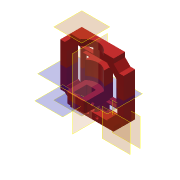
# Autodesk Inventor part: 20_Cube_Inser_Flexuremanipulator_ST_connector_zonly_v3
Saved by Autodesk Inventor 2019.4 (Build 234330000, 330)
## iProperties
Created: 2019-07-01
Part Number: 20_Cube_Inser_Flexuremanipulator_ST_connector_zonly_v3
Material: Generic
Document SubType Name: Modeling
Designer: diederichbenedict
Density: 1 g/cm^3
Appearance: Light Red
Author: diederichbenedict
Autodesk Inventor part; units mm, degrees
ref_plane "YZ Plane" through (0, 0, 0) normal (1, 0, 0) x (0, 1, 0)
ref_plane "XZ Plane" through (0, 0, 0) normal (0, 1, 0) x (-1, 0, 0)
ref_plane "Work Plane1" through (0, 0, 10) normal (0, 0, 1) x (1, 0, 0)
ref_plane "Work Plane4" through (0, 0, 13) normal (0, 0, 1) x (1, 0, 0)
sketch "Sketch5" plane through (0, 0, 13) normal (0, 0, 1) x (1, 0, 0)
  line L0 (-3.9299, 45.8299) -> (-37.9299, 45.8299) projected
  line L1 (-37.9299, 45.8299) -> (-37.9299, 42.2551) projected
  line L2 (-37.9299, 42.2551) -> (-42.2551, 37.9299) projected
  line L3 (-42.2551, 37.9299) -> (-45.8299, 37.9299) projected
  line L4 (-45.8299, 37.9299) -> (-45.8299, 3.9299) projected
  line L5 (-42.2551, 3.9299) -> (-45.8299, 3.9299) projected
  line L6 (-37.9299, -0.3953) -> (-42.2551, 3.9299) projected
  line L7 (-37.9299, -3.9701) -> (-37.9299, -0.3953) projected
  line L8 (-3.9713, -3.9701) -> (-37.9299, -3.9701) projected
  line L9 (-3.9713, -3.9701) -> (-3.9713, -0.4367) projected
  line L10 (-3.9713, -0.4367) -> (0.3953, 3.9299) projected
  line L11 (0.3953, 3.9299) -> (3.9701, 3.9299) projected
  line L12 (3.9701, 3.9299) -> (3.9701, 37.9299) projected
  line L13 (3.9701, 37.9299) -> (0.3953, 37.9299) projected
  line L14 (0.3953, 37.9299) -> (-3.9299, 42.2551) projected
  line L15 (-3.9299, 42.2551) -> (-3.9299, 45.8299) projected
  line L16 (-1.0299, 32.9299) -> (-1.0299, 8.9299)
  line L17 (-1.0299, 8.9299) -> (-1.6758, 8.9299)
  line L18 (-1.6758, 8.9299) -> (-8.9713, 1.6344)
  line L19 (-8.9713, 1.6344) -> (-8.9713, 1.0299)
  line L20 (-8.9713, 1.0299) -> (-32.9299, 1.0299)
  line L21 (-32.9299, 1.0299) -> (-32.9299, 1.6758)
  line L22 (-32.9299, 1.6758) -> (-40.184, 8.9299)
  line L23 (-40.184, 8.9299) -> (-40.8299, 8.9299)
  line L24 (-40.8299, 8.9299) -> (-40.8299, 32.9299)
  line L25 (-40.8299, 32.9299) -> (-40.184, 32.9299)
  line L26 (-40.184, 32.9299) -> (-32.9299, 40.184)
  line L27 (-32.9299, 40.184) -> (-32.9299, 40.8299)
  line L28 (-32.9299, 40.8299) -> (-8.9299, 40.8299)
  line L29 (-8.9299, 40.8299) -> (-8.9299, 40.184)
  line L30 (-8.9299, 40.184) -> (-1.6758, 32.9299)
  line L31 (-1.6758, 32.9299) -> (-1.0299, 32.9299)
  dimension "d46" = 5
  constraints: 32 end point, 15 other
  measures "d46" distance between parallel lines of L12 L16
extrude "Extrusion5" add sketch "Sketch5" along normal blind 6 and the other way blind 3
ref_plane "Work Plane5" through (0, 0, 21) normal (0, 0, 1) x (1, 0, 0)
sketch "Sketch7" plane through (0, 0, 10) normal (0, 0, 1) x (1, 0, 0)
  line L0 (-1.0299, 8.9299) -> (-1.6758, 8.9299) projected
  line L1 (-1.6758, 8.9299) -> (-8.9713, 1.6344) projected
  line L2 (-8.9713, 1.6344) -> (-8.9713, 1.0299) projected
  line L3 (-8.9713, 1.0299) -> (-32.9299, 1.0299) projected
  line L4 (-32.9299, 1.0299) -> (-32.9299, 1.6758) projected
  line L5 (-32.9299, 1.6758) -> (-40.184, 8.9299) projected
  line L6 (-40.184, 8.9299) -> (-40.8299, 8.9299) projected
  line L7 (-40.8299, 8.9299) -> (-40.8299, 32.9299) projected
  line L8 (-40.8299, 32.9299) -> (-40.184, 32.9299) projected
  line L9 (-40.184, 32.9299) -> (-32.9299, 40.184) projected
  line L10 (-32.9299, 40.184) -> (-32.9299, 40.8299) projected
  line L11 (-32.9299, 40.8299) -> (-8.9299, 40.8299) projected
  line L12 (-8.9299, 40.8299) -> (-8.9299, 40.184) projected
  line L13 (-8.9299, 40.184) -> (-1.6758, 32.9299) projected
  line L14 (-1.6758, 32.9299) -> (-1.0299, 32.9299) projected
  line L15 (-1.0299, 32.9299) -> (-1.0299, 8.9299) projected
  line L16 (-3.9299, 45.8299) -> (-37.9299, 45.8299) projected
  line L17 (-37.9299, 45.8299) -> (-37.9299, 42.2551) projected
  line L18 (-37.9299, 42.2551) -> (-42.2551, 37.9299) projected
  line L19 (-42.2551, 37.9299) -> (-45.8299, 37.9299) projected
  line L20 (-45.8299, 37.9299) -> (-45.8299, 3.9299) projected
  line L21 (-45.8299, 3.9299) -> (-42.2551, 3.9299) projected
  line L22 (-42.2551, 3.9299) -> (-37.9299, -0.3953) projected
  line L23 (-37.9299, -0.3953) -> (-37.9299, -3.9701) projected
  line L24 (-37.9299, -3.9701) -> (-3.9713, -3.9701) projected
  line L25 (-3.9713, -3.9701) -> (-3.9713, -0.4367) projected
  line L26 (-3.9713, -0.4367) -> (0.3953, 3.9299) projected
  line L27 (0.3953, 3.9299) -> (3.9701, 3.9299) projected
  line L28 (3.9701, 3.9299) -> (3.9701, 37.9299) projected
  line L29 (3.9701, 37.9299) -> (0.3953, 37.9299) projected
  line L30 (0.3953, 37.9299) -> (-3.9299, 42.2551) projected
  line L31 (-3.9299, 42.2551) -> (-3.9299, 45.8299) projected
  line L32 (-26.9299, 32.9299) -> (-26.9299, 16.9299)
  arc A0 (-40.8299, 32.9299) -> (-26.9299, 32.9299) centre (-33.8799, 32.9299) ccw construction
  arc A1 (-40.8299, 31.9299) -> (-26.9299, 31.9299) centre (-33.8799, 32.9299) ccw construction
  line L33 (-26.9299, 31.9299) -> (-40.8299, 31.9299) construction
  line L34 (-40.8299, 32.9299) -> (-40.8299, 31.9299)
  line L35 (-26.9299, 31.9299) -> (-26.9299, 32.9299)
  line L36 (-26.9299, 16.9299) -> (-26.9299, 17.9299)
  arc A2 (-40.8299, 16.9299) -> (-26.9299, 16.9299) centre (-33.8799, 17.9299) ccw construction
  line L37 (-26.9299, 16.9299) -> (-40.8299, 16.9299) construction
  line L38 (-40.8299, 17.9299) -> (-40.8299, 16.9299)
  arc A3 (-40.8299, 17.9299) -> (-26.9299, 17.9299) centre (-33.8799, 17.9299) ccw construction
  line L39 (-28.4506, 9.9466) -> (-20.9506, 9.9466)
  line L40 (-20.9506, 9.9466) -> (-20.9506, 31.9466)
  line L41 (-20.9506, 31.9466) -> (-28.4506, 31.9466)
  line L42 (-28.4506, 31.9466) -> (-28.4506, 9.9466)
  point P0 (-39.7698, 31.9299)
  point P1 (-39.8299, 31.9299)
  point P2 (-40.184, 17.9299)
  point P3 (-39.7698, 16.9299)
  point P4 (-39.8299, 16.9299)
  dimension "d55" = 15
  dimension "d176" = 23.9586
  dimension "d177" = 11.9793
  dimension "d178" = 7.5
  dimension "d179" = 22
  constraints: 22 end point, 10 point on circle, 4 centre point, 2 concentric, 2 parallel, 1 collinear, 1 horizontal, 1 perpendicular, 1 point on line, 1 vertical, 15 other
  measures "d55" distance of L7.end A3.start
  measures "d176" distance between parallel lines of L2 L4
  measures "d177" distance from line of L40 L4.end
  measures "d178" distance between parallel lines of L42 L40
  measures "d179" distance between parallel lines of L41 L39
extrude "Extrusion6" add sketch "Sketch7" along normal up to surface (9 mm away) contours L42 L41 L40 L39
sketch "Sketch10" plane through (0, 0, 19) normal (0, 0, 1) x (1, 0, 0)
  line L0 (-23.8799, 19.844) -> (-20.9799, 19.844) projected
  line L1 (-28.4506, 17.9466) -> (-20.9506, 17.9466)
  line L2 (-20.9506, 17.9466) -> (-20.9506, 9.9466)
  line L3 (-20.9506, 9.9466) -> (-28.4506, 9.9466)
  line L4 (-28.4506, 9.9466) -> (-28.4506, 17.9466)
  line L5 (-20.9506, 31.9466) -> (-20.9506, 9.9466) projected
  point P0 (0, 0)
  point P1 (-39.8299, 28.4889)
  point P2 (-2.0299, 28.4889)
  dimension "d140" = 8
  constraints: 8 end point, 2 parallel, 1 coincident, 1 horizontal, 1 perpendicular, 1 point on line
  measures "d140" distance of L1.end L2.end
extrude "Extrusion9" add sketch "Sketch10" along normal blind 13
ref_plane "Work Plane8" through (-37.9299, 45.8299, 10) normal (0, 1, 0) x (1, 0, 0)
ref_plane "Work Plane3" through (-27.93, 13.0477, 35) normal (0, -1, 0) x (1, 0, 0)
sketch "Sketch19" plane through (0, 0, 19) normal (0, 0, 1) x (1, 0, 0)
  line L0 (-23.3799, -3.9701) -> (-23.3799, 2.0299) projected
  line L1 (-18.4799, -3.9701) -> (-18.4799, 2.0299) projected
  circle A0 centre (-24.6083, -0.7296) radius 1.45
  circle A1 centre (-17.2627, -0.7296) radius 1.45
  point P0 (0, 0)
  dimension "d109" = 2.9
  dimension "d110" = 2.9
  constraints: 2 centre point
  measures "d109" diameter of A0
  measures "d110" diameter of A1
extrude "Extrusion17" cut sketch "Sketch19" against normal blind 7
sketch "Sketch20" plane through (0, 0, 10) normal (0, 0, -1) x (-1, 0, 0)
  line L0 (25.9299, 9.9299) -> (15.9299, 9.9299) projected
  line L1 (25.9299, 31.9299) -> (25.9299, 9.9299) projected
  line L2 (15.9299, 31.9299) -> (25.9299, 31.9299) projected
  line L3 (15.9299, 9.9299) -> (15.9299, 31.9299) projected
  line L4 (15.9299, 9.9299) -> (15.9299, 31.9299) projected
  line L5 (15.9299, 34.4094) -> (15.9299, 35.1094)
  line L6 (7.7745, 34.5094) -> (7.7745, 35.0094)
  line L7 (1.9699, 29.7049) -> (1.9699, 12.1049) projected
  line L8 (39.8899, 12.1049) -> (39.8899, 29.7049) projected
  line L9 (32.9299, 1.0299) -> (8.9713, 1.0299) projected
  line L10 (15.9299, 31.9299) -> (25.9299, 31.9299) projected
  line L11 (27.6381, 40.8299) -> (14.2217, 40.8299) projected
  line L12 (15.9299, 34.4094) -> (20.9299, 34.4094)
  line L13 (20.9299, 34.4094) -> (20.9299, 40.8299)
  line L14 (20.9299, 40.8299) -> (15.9299, 40.8299)
  line L15 (15.9299, 40.8299) -> (15.9299, 34.4094)
  line L16 (15.9299, 27.9299) -> (15.9299, 31.9299)
  line L17 (5.7745, 31.9299) -> (7.7745, 31.9299)
  line L18 (7.7745, 31.9299) -> (7.7745, 35.0094)
  line L19 (7.7745, 35.0094) -> (5.7745, 35.0094)
  line L20 (5.7745, 35.0094) -> (5.7745, 31.9299)
  line L21 (20.9299, 34.4094) -> (15.9299, 34.4094)
  line L22 (15.9299, 34.4094) -> (15.9299, 33.9799)
  line L23 (5.7745, 35.0094) -> (7.7745, 35.0094)
  line L24 (15.9299, 53.9299) -> (15.9299, 31.9299)
  line L25 (15.9299, 53.9299) -> (15.9299, 31.9299)
  line L26 (15.9299, 29.4504) -> (15.9299, 28.7504)
  line L27 (7.7745, 29.3504) -> (7.7745, 28.8504)
  line L28 (15.9299, 35.9299) -> (15.9299, 31.9299)
  line L29 (7.7745, 31.9299) -> (7.7745, 28.8504)
  line L30 (5.7745, 28.8504) -> (5.7745, 31.9299)
  line L31 (20.9299, 29.4504) -> (15.9299, 29.4504)
  line L32 (15.9299, 29.4504) -> (15.9299, 29.8799)
  line L33 (7.7745, 28.8504) -> (7.7745, 28.8504)
  line L34 (5.7745, 28.8504) -> (5.7745, 28.8504)
  line L35 (7.7745, 28.8504) -> (7.7745, 20.9299)
  line L36 (7.7745, 20.9299) -> (5.7745, 20.9299)
  line L37 (5.7745, 20.9299) -> (5.7745, 28.8504)
  line L38 (15.9299, 34.4094) -> (7.7745, 34.4094)
  line L39 (7.7745, 34.4094) -> (7.7745, 35.0094)
  line L40 (7.7745, 35.0094) -> (15.9299, 35.0094)
  line L41 (15.9299, 35.0094) -> (15.9299, 34.4094)
  line L42 (7.7745, 32.0299) -> (7.7745, 31.4299)
  line L43 (15.9299, 31.4299) -> (15.9299, 31.9299)
  line L44 (15.9299, 31.9299) -> (15.9299, 19.844) projected
  line L45 (7.7745, 31.9299) -> (15.9299, 31.9299)
  line L46 (15.9299, 31.9299) -> (15.9299, 31.3299)
  line L47 (15.9299, 31.3299) -> (7.7745, 31.3299)
  line L48 (7.7745, 31.3299) -> (7.7745, 31.9299)
  point P0 (0, 0)
  dimension "d151" = 0
  dimension "d152" = 0
  dimension "d162" = 0
  dimension "d163" = 2
  dimension "d165" = 0.6
  dimension "d166" = 0
  dimension "d188" = 0.6
  constraints: 76 end point, 11 symmetric about line, 10 parallel, 6 horizontal, 5 perpendicular, 2 point on line, 1 midpoint, 2 other
  measures "d151" distance between parallel lines of L3 L15
  measures "d152" distance between parallel lines of L5 L22
  measures "d162" distance between parallel lines of L30 L37
  measures "d163" distance between parallel lines of L37 L35
  measures "d165" distance of L45.end L46.end
  measures "d166" distance between parallel lines of L2 L45
  measures "d188" distance between parallel lines of L38 L40
extrude "Extrusion18" add sketch "Sketch20" against normal blind 3 contours L0 L3 L2 L1 | L3 L47 L29 L45 | L29 L27 L35 L36 L37 L30 L17 | L17 L20 L19 L6 L18 | L38 L18 L6 L40 L5 | L5 L15 L11 L13 L12
ref_plane "Work Plane9" through (-20.9299, 3.9299, 19) normal (1, 0, 0) x (0, 0, -1)
ref_plane "Work Plane10" through (-37.9299, 20.9299, 19) normal (0, -1, 0) x (1, 0, 0)
mirror "Mirror2" about plane through (-20.9299, 3.9299, 19) normal (1, 0, 0) of "Extrusion18", "Extrusion6", "Extrusion9"
mirror "Mirror3" about plane through (-37.9299, 20.9299, 19) normal (0, -1, 0) of "Extrusion18", "Mirror2"
ref_plane "Work Plane11" through (-37.9299, -3.9701, 10) normal (0, -1, 0) x (1, 0, 0)
sketch "Sketch8" plane through (-37.9299, -3.9701, 10) normal (0, -1, 0) x (1, 0, 0)
  line L0 (12.756, 11) -> (21.244, 11) projected
  line L1 (12.756, 4) -> (21.244, 4) projected
  circle A0 centre (17, 5.6001) radius 2.45
  line L2 (21.244, 11) -> (21.244, 4) projected
  line L3 (12.756, 4) -> (12.756, 11) projected
  point P0 (37.9299, -10)
  dimension "d67" = 4.9
  constraints: 1 centre point
  measures "d67" diameter of A0
extrude "Extrusion7" cut sketch "Sketch8" against normal blind 7 contours A0 L1 | L1 A0
sketch "Sketch21" plane through (-37.9299, 45.8299, 19) normal (0, 1, 0) x (1, 0, 0)
  circle A0 centre (16.9, -6.047) radius 2.9 projected
  line L0 (12, 0) -> (22, 0) projected
  line L1 (12, 0) -> (12, -11) projected
  line L2 (22, -11) -> (12, -11) projected
  line L3 (22, 0) -> (22, -11) projected
  circle A1 centre (16.9, -6.047) radius 11
  point P0 (37.9299, 19)
  dimension "d137" = 22
  constraints: 1 centre point, 1 coincident
  measures "d137" diameter of A1
extrude "Extrusion19" cut sketch "Sketch21" against normal up to surface (27.8834 mm away) contours A0 | L0 L3 L2 L1 | A1
sketch "Sketch27" plane through (-28.4506, 9.9466, 32) normal (0, -1, 0) x (1, 0, 0)
  line L0 (10.8707, -12.053) -> (10.8707, -2.953) projected
  arc A0 (10.8707, -2.953) -> (10.3707, -2.453) centre (10.3707, -2.953) ccw projected
  line L1 (10.3707, -2.453) -> (4.4707, -2.453) projected
  arc A1 (4.4707, -2.453) -> (3.9707, -2.953) centre (4.4707, -2.953) ccw projected
  line L2 (3.9707, -2.953) -> (3.9707, -12.053) projected
  arc A2 (3.9707, -12.053) -> (4.4707, -12.553) centre (4.4707, -12.053) ccw projected
  line L3 (4.4707, -12.553) -> (10.3707, -12.553) projected
  arc A3 (10.3707, -12.553) -> (10.8707, -12.053) centre (10.3707, -12.053) ccw projected
  line L4 (8.2707, -4.303) -> (8.2707, -3.753) projected
  line L5 (9.7207, -4.303) -> (8.2707, -4.303) projected
  line L6 (9.7207, -8.903) -> (9.7207, -4.303) projected
  line L7 (9.0707, -8.903) -> (9.7207, -8.903) projected
  line L8 (9.0707, -9.703) -> (9.0707, -8.903) projected
  line L9 (9.7207, -9.703) -> (9.0707, -9.703) projected
  line L10 (9.7207, -10.803) -> (9.7207, -9.703) projected
  line L11 (8.7207, -10.803) -> (9.7207, -10.803) projected
  line L12 (8.7207, -11.803) -> (8.7207, -10.803) projected
  line L13 (6.1207, -11.803) -> (8.7207, -11.803) projected
  line L14 (6.1207, -10.803) -> (6.1207, -11.803) projected
  line L15 (5.1207, -10.803) -> (6.1207, -10.803) projected
  line L16 (5.1207, -9.703) -> (5.1207, -10.803) projected
  line L17 (5.7707, -9.703) -> (5.1207, -9.703) projected
  line L18 (5.7707, -8.903) -> (5.7707, -9.703) projected
  line L19 (5.1207, -8.903) -> (5.7707, -8.903) projected
  line L20 (5.1207, -4.303) -> (5.1207, -8.903) projected
  line L21 (6.5707, -4.303) -> (5.1207, -4.303) projected
  line L22 (6.5707, -3.753) -> (6.5707, -4.303) projected
  line L23 (8.2707, -3.753) -> (6.5707, -3.753) projected
  line L24 (4.4707, -2.253) -> (10.3707, -2.253)
  arc A4 (11.0707, -2.953) -> (10.3707, -2.253) centre (10.3707, -2.953) ccw
  line L25 (11.0707, -2.953) -> (11.0707, -12.053)
  arc A5 (10.3707, -12.753) -> (11.0707, -12.053) centre (10.3707, -12.053) ccw
  line L26 (10.3707, -12.753) -> (4.4707, -12.753)
  arc A6 (3.7707, -12.053) -> (4.4707, -12.753) centre (4.4707, -12.053) ccw
  line L27 (3.7707, -12.053) -> (3.7707, -2.953)
  arc A7 (4.4707, -2.253) -> (3.7707, -2.953) centre (4.4707, -2.953) ccw
  point P0 (28.4506, -32)
  dimension "d183" = 0.2
  constraints: 8 end point, 8 point on circle, 4 centre point, 7 other
  measures "d183" distance between parallel lines of L1 L24
extrude "Extrusion25" cut sketch "Sketch27" against normal up to surface (8 mm away) contours A3 L3 A2 L2 A1 L1 A0 L0 | L5 L6 L7 L8 L9 L10 L11 L12 L13 L14 L15 L16 L17 L18 L19 L20 L21 L22 L23 L4 | L24 A4 L25 A5 L26 A6 L27 A7
fillet "Fillet4" radius 2 2 edges at (-13.4092, 13.9466, 32) (-28.4506, 13.9466, 32)
sketch "Sketch28" plane through (-28.4506, 31.9299, 10) normal (-1, 0, 0) x (0, 0, 1)
  circle A0 centre (15.9248, -18.0684) radius 1.4
  point P0 (-10, -31.9299)
  dimension "d185" = 2.8
  constraints: 1 centre point
  measures "d185" diameter of A0
extrude "Extrusion26" cut sketch "Sketch28" against normal through all
body "Solid1"
